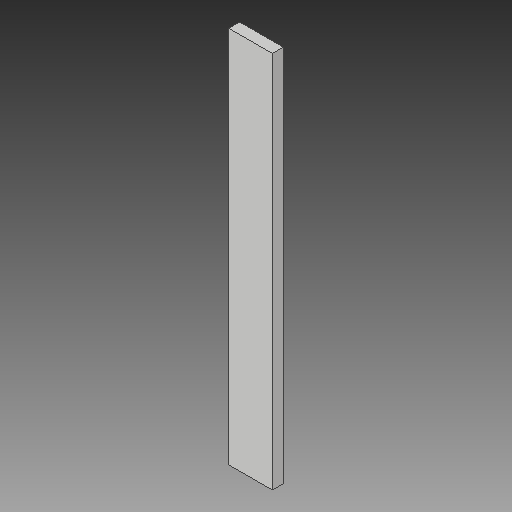
# Autodesk Inventor part: CollectionPost
Saved by Autodesk Inventor 2019 (Build 230136000, 136)
## iProperties
Created: 2018-11-10
Part Number: CollectionPost
Material: Generic
Document SubType Name: Modeling
Designer: User
Density: 1 g/cm^3
Appearance: Default
Author: User
Autodesk Inventor part; units mm, degrees
ref_plane "YZ Plane" through (0, 0, 0) normal (1, 0, 0) x (0, 1, 0)
ref_plane "XZ Plane" through (0, 0, 0) normal (0, 1, 0) x (-1, 0, 0)
ref_plane "XY Plane" through (0, 0, 0) normal (0, 0, 1) x (1, 0, 0)
sketch "Sketch1" plane through (0, 0, 0) normal (0, 0, 1) x (1, 0, 0)
  line L0 (0, 0) -> (38.1, 0)
  line L1 (38.1, 0) -> (38.1, 330.2)
  line L2 (38.1, 330.2) -> (0, 330.2)
  line L3 (0, 330.2) -> (0, 0)
  dimension "d0" = 38.1
  dimension "d1" = 330.2
  constraints: 8 end point, 2 parallel, 1 horizontal, 1 perpendicular
  measures "d0" distance of L2.end L1.end
  measures "d1" distance of L1.end L0.end
extrude "Extrusion1" add sketch "Sketch1" along normal blind 9.525
sketch "Sketch2" plane through (0, 0, 0) normal (0, -1, 0) x (1, 0, 0)
  line L0 (0, 0) -> (38.1, 0) projected
  line L1 (38.1, 0) -> (38.1, 9.525) projected
  line L2 (0, 9.525) -> (38.1, 9.525) projected
  line L3 (0, 0) -> (0, 9.525) projected
  point P0 (31.75, 4.7625)
  point P1 (6.35, 4.7625)
  dimension "d4" = 25.4
  dimension "d5" = 38.1
  dimension "d6" = 9.525
  dimension "d7" = 6.35
  dimension "d8" = 4.7625
  dimension "d9" = 4.7625
  measures "d4" distance of point (6.35, 4.762) point (31.75, 4.763)
  measures "d5" distance of L2.start L1.end
  measures "d6" distance of L0.end L1.end
  measures "d7" distance from line of L1 point (31.75, 4.763)
  measures "d8" distance from line of L2 point (6.35, 4.762)
  measures "d9" distance from line of L2 point (31.75, 4.763)
hole "Hole1" at (31.75, 0, 4.7625) at (6.35, 0, 4.7625) direction (0, 1, 0) diameter 3.683 depth 25.4 tip angle 118 thread size "10-24 UNC" class "2B" standard "ANSI Unified Screw Threads"
equation "\"d8\" = 0.5 * d6"
equation "\"d9\" = d8"
body "Solid1"
